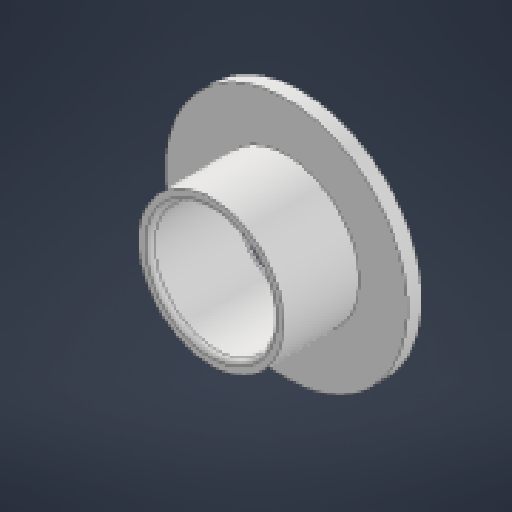
# Autodesk Inventor part: M3Spacer
Saved by Autodesk Inventor 2024.1 (Build 281209000, 209)
## iProperties
Created: 2023-11-14
Part Number: M3Spacer
Material: Generic
Document SubType Name: Modeling
Designer: Brandon
Density: 1 g/cm^3
Appearance: Default
Author: Brandon
Autodesk Inventor part; units mm, degrees
ref_plane "YZ Plane" through (0, 0, 0) normal (1, 0, 0) x (0, 1, 0)
ref_plane "XZ Plane" through (0, 0, 0) normal (0, 1, 0) x (-1, 0, 0)
ref_plane "XY Plane" through (0, 0, 0) normal (0, 0, 1) x (1, 0, 0)
sketch "Sketch1" plane through (0, 0, 0) normal (0, 0, 1) x (1, 0, 0)
  circle A0 centre (7.161, 8.0403) radius 1.524 projected
  line L0 (16.461, -12.7743) -> (16.461, -7.3635) projected
  arc A1 (16.461, -7.3635) -> (16.2925, -6.0336) centre (11.127, -7.3635) ccw projected
  line L1 (16.2925, -6.0336) -> (12.3265, 9.3703) projected
  arc A2 (12.3265, 9.3703) -> (7.161, 13.3743) centre (7.161, 8.0403) ccw projected
  line L2 (7.161, 13.3743) -> (-11.127, 13.3743) projected
  arc A3 (-11.127, 13.3743) -> (-16.461, 8.0403) centre (-11.127, 8.0403) ccw projected
  line L3 (-16.461, 8.0403) -> (-16.461, -8.0403) projected
  arc A4 (-16.461, -8.0403) -> (-11.127, -13.3743) centre (-11.127, -8.0403) ccw projected
  line L4 (-11.127, -13.3743) -> (15.861, -13.3743) projected
  arc A5 (15.861, -13.3743) -> (16.461, -12.7743) centre (15.861, -12.7743) ccw projected
  circle A6 centre (-11.127, 8.0403) radius 4.064 projected
  circle A7 centre (7.161, 8.0403) radius 1.6002
  circle A8 centre (7.161, 8.0403) radius 2.032 projected
  circle A9 centre (7.161, 8.0403) radius 1.905
  point P0 (0, 0)
  dimension "d0" = 0.0762
  dimension "d1" = 0.127
  constraints: 2 centre point
  measures "d0" radial gap between concentric circles of A0 A7
  measures "d1" radial gap between concentric circles of A8 A9
extrude "Extrusion1" add sketch "Sketch1" along normal blind 2.3495 contours A9
fillet "Fillet1" radius 0.127 2 edges at (5.5608, 8.0403, 2.3495) (5.5608, 8.0403, 0)
sketch "Sketch2" plane through (7.161, 8.0403, 0) normal (0, 0, -1) x (-1, 0, 0)
  circle A0 centre (0, 0) radius 1.905 projected
  circle A1 centre (0, 0) radius 3.175
  point P0 (7.161, -8.0403)
  dimension "d5" = 6.35
  constraints: 1 centre point, 1 coincident
  measures "d5" diameter of A1
extrude "Extrusion2" add sketch "Sketch2" against normal blind 0.381
body "Solid1"
